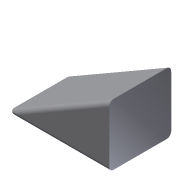
# Autodesk Inventor part: wedge mount
Saved by Autodesk Inventor 2012 (Build 160160000, 160)
## iProperties
Created: 2012-04-25
Part Number: wedge mount
Material: Default
Document SubType Name: Modeling
Designer: Antonella Wilby
Density: 1 g/cm^3
Author: Antonella Wilby
Autodesk Inventor part; units mm, degrees
ref_plane "YZ Plane" through (0, 0, 0) normal (1, 0, 0) x (0, 1, 0)
ref_plane "XZ Plane" through (0, 0, 0) normal (0, 1, 0) x (-1, 0, 0)
ref_plane "XY Plane" through (0, 0, 0) normal (0, 0, 1) x (1, 0, 0)
sketch "Sketch1" plane through (0, 0, 0) normal (0, 0, 1) x (1, 0, 0)
  line L0 (-106.68, 0) -> (106.68, 0) projected
  line L1 (0, -61.5917) -> (0, 61.5917) projected
  line L2 (76.2, 43.9941) -> (-76.2, -43.9941)
  line L3 (-76.2, -43.9941) -> (76.2, -43.9941)
  line L4 (76.2, -43.9941) -> (76.2, 43.9941)
  point P0 (0, 0)
  point P1 (0, -43.9941)
  point P2 (76.2, 0)
  dimension "d0" = 30
  dimension "d1" = 152.4
  constraints: 6 end point, 2 midpoint, 2 perpendicular, 1 horizontal alignment, 1 vertical alignment
  measures "d0" angle of L2 L3
  measures "d1" distance of L2.end L3.end
extrude "Extrusion1" add sketch "Sketch1" along normal mid plane 88.9
fillet "Fillet1" radius 3.175 1 edges at (-76.2, -43.9941, 0)
fillet "Fillet2" radius 6.35 6 edges at (-67.4176, -41.6408, 44.45) (5.9246, -43.9941, 44.45) (5.1309, 2.9623, 44.45) (-67.4176, -41.6408, -44.45) (5.9246, -43.9941, -44.45) (5.1309, 2.9623, -44.45)
body "Solid1"
